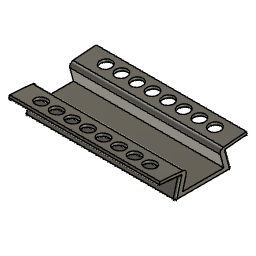
PCRtubeMagnetHolder v1 (Autodesk Fusion 360 design; units mm, degrees)
Autodesk Fusion 360 part; units mm, degrees
sketch "Sketch1" plane through (0, 0, 0) normal (1, 0, 0) x (0, 1, 0)
  line L0 (15.3146, 0) -> (15.3146, 3)
  line L1 (15.3146, 3) -> (26.5646, 3)
  line L2 (26.5646, 3) -> (23.9764, 12.6593)
  line L3 (26.5646, 3) -> (36.5646, 3) construction
  line L4 (23.9764, 12.6593) -> (38.9193, 13.9666)
  line L5 (23.9764, 12.6593) -> (38.9764, 12.6593) construction
  line L6 (38.9193, 13.9666) -> (39.5664, 11.5518)
  line L7 (31, 0) -> (28.1718, 10.5549)
  line L8 (39.5664, 11.5518) -> (28.1718, 10.5549)
  line L9 (31, 0) -> (15.3146, 0)
  dimension "d1" = 31
  dimension "d2" = 3
  dimension "d4" = 11.25
  dimension "d7" = 105
  dimension "d8" = 10
  dimension "d9" = 5
  dimension "d10" = 15
  dimension "d11" = 2.5
  constraint perpendicular L0 L1
  constraint horizontal L3
  constraint horizontal L5
  constraint parallel L2 L6
  constraint parallel L2 L7
  constraint parallel L4 L8
  constraint perpendicular L0 L9
  measures "d1" distance of origin L7.start
  measures "d2" distance of L0.start L0.end
  measures "d4" distance of L0.end L1.end
  measures "d7" angle of L2 L3
  measures "d8" distance of L1.end L2.end
  measures "d9" angle of L4 L5
  measures "d10" distance of L2.end L4.end
  measures "d11" distance of L4.end L6.end
extrude "Extrude1" add sketch "Sketch1" against normal blind 82
sketch "Sketch3" plane through (0, -0.917, 10.4814) normal (0, -0.087156, 0.996195) x (1, 0, 0)
  line L0 (0, 24.9885) -> (0, 39.9885)
  line L1 (0, 39.9885) -> (-82, 39.9885)
  line L2 (-82, 39.9885) -> (-82, 24.9885)
  line L3 (-82, 24.9885) -> (0, 24.9885)
  line L4 (-82, 39.9885) -> (-82, 33.9885) construction
  line L5 (-82, 33.9885) -> (0, 33.9885)
  circle A0 centre (-70.75, 33.9885) radius 3.25
  circle A1 centre (-45.25, 33.9885) radius 3.25
  circle A2 centre (-53.75, 33.9885) radius 3.25
  circle A3 centre (-62.25, 33.9885) radius 3.25
  circle A4 centre (-11.25, 33.9885) radius 3.25
  circle A5 centre (-19.75, 33.9885) radius 3.25
  circle A6 centre (-28.25, 33.9885) radius 3.25
  circle A7 centre (-36.75, 33.9885) radius 3.25
  dimension "d21" = 6
  dimension "d31" = 6.5
  dimension "d34" = 6.5
  dimension "d35" = 6.5
  dimension "d37" = 8.5
  dimension "d39" = 6.5
  dimension "d43" = 6.5
  dimension "d44" = 6.5
  dimension "d45" = 6.5
  dimension "d46" = 6.5
  dimension "d47" = 8.5
  dimension "d48" = 8.5
  dimension "d49" = 8.5
  dimension "d50" = 8.5
  dimension "d52" = 8.5
  dimension "d53" = 8.5
  dimension "d55" = 11.25
  dimension "d57" = 11.25
  constraint coincident L1.end L2.start
  constraint perpendicular L1 L4
  constraint coincident L0 L5.end
  constraint perpendicular L0 L5
  measures "d21" distance of L1.end L4.end
  measures "d31" diameter of A0
  measures "d34" diameter of A1
  measures "d37" distance of A1.centre A2.centre
  measures "d39" diameter of A3
  measures "d43" diameter of A7
  measures "d44" diameter of A6
  measures "d45" diameter of A4
  measures "d46" diameter of A5
  measures "d47" distance of A4.centre A5.centre
  measures "d48" distance of A1.centre A7.centre
  measures "d49" distance of A7.centre A6.centre
  measures "d50" distance of A6.centre A5.centre
  measures "d52" distance of A2.centre A3.centre
  measures "d53" distance of A0.centre A3.centre
  measures "d55" distance of L4 A0.centre
  measures "d57" distance of L5.end A4.centre
extrude "Extrude2" cut sketch "Sketch3" against normal blind 2.5 contours L5 A4 | L5 A4 | L5 A0 | L5 A0 | L5 A5 | L5 A5 | L5 A3 | L5 A3 | L5 A6 | L5 A6 | L5 A2 | L5 A2 | L5 A7 | L5 A7 | L5 A1 | L5 A1
mirror "Mirror1" about plane through (0, 15.3146, 0) normal (0, -1, 0) of bodies 1 merged
fillet "Fillet1" radius 1 16 edges at (-65.2801, 31.9859, 10.8886) (-73.7801, 31.9859, 10.8886) (-56.7801, 31.9859, 10.8886) (-48.2801, 31.9859, 10.8886) (-39.7801, 31.9859, 10.8886) (-22.7801, 31.9859, 10.8886) (-31.2801, 31.9859, 10.8886) (-14.2801, 31.9859, 10.8886) (-14.2801, -1.3568, 10.8886) (-22.7801, -1.3568, 10.8886) (-39.7801, -1.3568, 10.8886) (-31.2801, -1.3568, 10.8886) (-48.2801, -1.3568, 10.8886) (-56.7801, -1.3568, 10.8886) (-65.2801, -1.3568, 10.8886) (-73.7801, -1.3568, 10.8886)
fillet "Fillet2" radius 1 11 edges at (-82, -3.2399, 11.0533) (-41, -8.9372, 11.5518) (-82, 1.0433, 5.2774) (-82, 15.3146, 0) (-82, 29.5859, 5.2774) (-82, 33.8691, 11.0533) (-41, 39.5664, 11.5518) (-41, 31, 0) (0, 15.3146, 0) (0, 29.5859, 5.2774) (0, 33.8691, 11.0533)
fillet "Fillet2" radius 1 3 edges at (-41, -0.3708, 0) (0, 1.0433, 5.2774) (0, -3.2399, 11.0533)
fillet "Fillet2" radius 2 2 edges at (-41, 6.6528, 12.6593) (-41, 23.9764, 12.6593)
